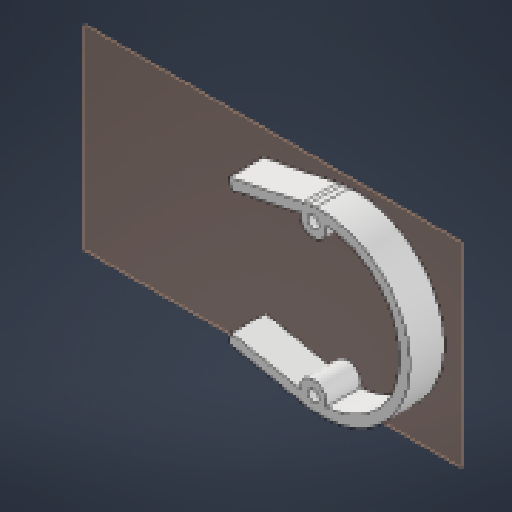
# Autodesk Inventor part: MotorCover
Saved by Autodesk Inventor 2024.2 (Build 282272000, 272)
## iProperties
Created: 2023-12-22
Part Number: MotorCover
Material: 一般
Document SubType Name: Modeling
Designer: Hanaoka
Density: 1 g/cm^3
Appearance: 既定
Author: Hanaoka
Autodesk Inventor part; units mm, degrees
ref_plane "YZ Plane" through (0, 0, 0) normal (1, 0, 0) x (0, 1, 0)
ref_plane "XZ Plane" through (0, 0, 0) normal (0, 1, 0) x (-1, 0, 0)
ref_plane "XY Plane" through (0, 0, 0) normal (0, 0, 1) x (1, 0, 0)
ref_plane "作業平面1" through (0, 0, 0) normal (0, 0, 1) x (1, 0, 0)
sketch "スケッチ1" plane through (0, 0, 0) normal (0, 0, 1) x (1, 0, 0)
  arc A0 (9.4, -12.7373) -> (9.4, 12.7373) centre (12, 0) ccw projected
  circle A1 centre (10.8888, 11) radius 0.8 projected
  circle A2 centre (10.8888, -11) radius 0.8 projected
  circle A3 centre (10.8888, 11) radius 2
  circle A4 centre (10.8888, -11) radius 2
  arc A5 (12.8328, -11.4698) -> (12.8328, 11.4698) centre (12, 0) ccw
  line L0 (9.4, 12.7373) -> (-19.4, 6.8586) projected
  line L1 (-19.4, -6.8586) -> (9.4, -12.7373) projected
  line L2 (-1.4086, 10.5311) -> (-1.1086, 9.0614)
  line L3 (-1.1086, 9.0614) -> (8.8914, 11.1026)
  line L4 (-1.4086, -10.5311) -> (-1.1086, -9.0614)
  line L5 (-1.1086, -9.0614) -> (8.8914, -11.1026)
  point P0 (0, 0)
  point P1 (10.1875, -12.873)
  point P2 (11.2013, -12.9754)
  point P3 (11.2013, 12.9754)
  point P4 (10.1875, 12.873)
  dimension "d0" = 4
  dimension "d1" = 1.5
  dimension "d2" = 1.5
  dimension "d3" = 10
  constraints: 8 end point, 6 point on circle, 3 centre point, 3 coincident, 3 perpendicular, 2 equal length, 2 point on line, 1 equal radius, 1 parallel
  measures "d0" diameter of A3
  measures "d1" radial gap between concentric circles of A0 A5
  measures "d2" distance between parallel lines of L0 L3
  measures "d3" horizontal distance of L2.end L3.end
extrude "押し出し1" add sketch "スケッチ1" along normal blind 5
